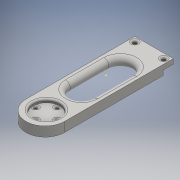
# Autodesk Inventor part: LowerArmPartAv2
Saved by Autodesk Inventor 2016 (Build 200138000, 138)
## iProperties
Created: 2015-10-06
Part Number: LowerArmPartAv2
Material: Generic
Document SubType Name: Modeling
Designer: alex
Density: 1 g/cm^3
Appearance: Default
Mass: 56.6565 g
Surface Area: 198.211 cm^2
Volume: 56.6565 cm^3
Author: alex
Autodesk Inventor part; units mm, degrees
ref_plane "YZ Plane" through (0, 0, 0) normal (1, 0, 0) x (0, 1, 0)
ref_plane "XZ Plane" through (0, 0, 0) normal (0, 1, 0) x (-1, 0, 0)
ref_plane "XY Plane" through (0, 0, 0) normal (0, 0, 1) x (1, 0, 0)
sketch "Sketch1" plane through (0, 0, 0) normal (0, 0, 1) x (1, 0, 0)
  line L0 (-20, 50) -> (20, 50)
  line L1 (20, 50) -> (20, -83)
  line L2 (20, -83) -> (-20, -83)
  line L3 (-20, -83) -> (-20, 50)
  point P0 (0, 0)
  dimension "d0" = 50
  dimension "d1" = 83
  dimension "d2" = 20
  dimension "d3" = 20
  constraints: 8 end point, 2 parallel, 1 horizontal, 1 perpendicular
  measures "d0" distance from line of point (0, 0) L0
  measures "d1" distance from line of point (0, 0) L2
  measures "d2" distance from line of point (0, 0) L3
  measures "d3" distance from line of point (0, 0) L1
extrude "Extrusion1" add sketch "Sketch1" along normal blind 10
sketch "Sketch6" plane through (0, 0, 10) normal (0, 0, 1) x (1, 0, 0)
  circle A0 centre (0, -61.75) radius 13.75
  arc A1 (-18, -63) -> (18, -63) centre (0, -63) ccw projected
  line L0 (18, 20) -> (18, -83) projected
  circle A2 centre (0, -50.5) radius 1.5
  circle A3 centre (-11.25, -61.75) radius 1.5
  circle A4 centre (0, -73) radius 1.5
  circle A5 centre (11.25, -61.75) radius 1.5
  line L1 (0, 0) -> (-53.5469, 0)
  dimension "d41" = 27.5
  dimension "d42" = 5.5
  dimension "d43" = 18
  dimension "d44" = 3
  dimension "d45" = 11.25
  dimension "d46" = 18
  dimension "d49" = 360
  constraints: 5 centre point, 2 end point, 1 horizontal, 9 other
  measures "d41" diameter of A0
  measures "d43" distance from line of L0 A0.centre
  measures "d44" diameter of A2
  measures "d45" distance of A0.centre A2.centre
  measures "d46" distance from line of L0 A2.centre
sketch "Sketch8" plane through (0, 0, 10) normal (0, 0, 1) x (1, 0, 0)
  circle A0 centre (0, -61.75) radius 13.75
  line L0 (-18, -83) -> (-18, 20) projected
  arc A1 (-18, -63) -> (18, -63) centre (0, -63) ccw projected
  line L1 (0, 0) -> (-37.1861, 0)
  dimension "d62" = 27.5
  dimension "d63" = 18
  dimension "d64" = 1.25
  constraints: 2 end point, 1 centre point, 1 horizontal
  measures "d62" diameter of A0
  measures "d63" distance from line of L0 A0.centre
  measures "d64" distance of A1.centre A0.centre
extrude "Extrusion8" cut sketch "Sketch8" against normal blind 3.5
fillet "Fillet12" radius 20 2 edges at (-20, -83, 5) (20, -83, 5)
sketch "Sketch10" plane through (0, 0, 10) normal (0, 0, 1) x (1, 0, 0)
  line L0 (0, 27) -> (0, -37) construction
  line L1 (-12, 15) -> (-12, -25)
  line L2 (12, -25) -> (12, 15)
  arc A0 (12, 15) -> (-12, 15) centre (0, 15) ccw
  arc A1 (-12, -25) -> (12, -25) centre (0, -25) ccw
  line L3 (20, 50) -> (-20, 50) projected
  line L4 (20, -63) -> (20, 50) projected
  line L5 (-20, 50) -> (-20, -63) projected
  point P0 (0, 0)
  point P1 (0, -5)
  dimension "d80" = 40
  dimension "d81" = 35
  dimension "d82" = 8
  dimension "d83" = 8
  constraints: 8 end point, 6 point on circle, 4 tangent, 2 centre point, 2 point on line, 1 midpoint, 1 parallel, 1 vertical
  measures "d80" distance of A1.centre A0.centre
  measures "d81" distance from line of L3 A0.centre
  measures "d82" distance between parallel lines of L4 L2
  measures "d83" distance between parallel lines of L5 L1
extrude "Extrusion10" cut sketch "Sketch10" against normal through all
sketch "Sketch11" plane through (0, 0, 10) normal (0, 0, 1) x (1, 0, 0)
  point P0 (0, 0)
extrude "Extrusion11" cut sketch "Sketch6" against normal through all contours A2 | A3 | A4 | A5
sketch "Sketch13" plane through (0, 0, 0) normal (0, 0, -1) x (-1, 0, 0)
  line L0 (20, -63) -> (20, 50) projected
  line L1 (-20, 50) -> (20, 50)
  line L2 (20, 50) -> (20, 39.5)
  line L3 (20, 39.5) -> (-20, 39.5)
  line L4 (-20, 39.5) -> (-20, 50)
  line L5 (20, 50) -> (-20, 50) projected
  point P0 (0, 0)
  dimension "d91" = 10.5
  dimension "d92" = 0
  dimension "d93" = 40
  constraints: 8 end point, 2 parallel, 1 horizontal, 1 perpendicular, 1 point on line
  measures "d91" distance between parallel lines of L3 L1
  measures "d92" distance between parallel lines of L5 L1
  measures "d93" distance between parallel lines of L0 L4
extrude "Extrusion13" cut sketch "Sketch13" against normal blind 5
sketch "Sketch14" plane through (0, 0, 5) normal (0, 0, -1) x (-1, 0, 0)
  circle A0 centre (-15, 45) radius 2
  line L0 (20, 39.5) -> (-20, 39.5) projected
  line L1 (-20, -63) -> (-20, 50) projected
  line L2 (0, 0) -> (0, 62.9691)
  circle A1 centre (15, 45) radius 2
  line L3 (-20, 50) -> (20, 50) projected
  dimension "d96" = 4
  dimension "d98" = 5
  dimension "d105" = 5
  constraints: 2 centre point, 2 end point, 1 symmetric about line, 1 vertical, 1 other
  measures "d96" diameter of A0
  measures "d98" distance from line of L1 A0.centre
  measures "d105" distance from line of L3 A0.centre
extrude "Extrusion14" cut sketch "Sketch14" against normal blind 10 contours A0 | A1
fillet "Fillet13" radius 5 8 edges at (0, -37, 10) (-12, -5, 10) (0, 27, 10) (12, -5, 10) (0, 27, 0) (-12, -5, 0) (0, -37, 0) (12, -5, 0)
fillet "Fillet14" radius 2 2 edges at (-13, 45, 10) (17, 45, 10)
fillet "Fillet15" radius 2 2 edges at (-13, 45, 5) (17, 45, 5)
fillet "Fillet16" radius 2 9 edges at (-13.75, -61.75, 10) (-1.5, -50.5, 6.5) (9.75, -61.75, 6.5) (-12.75, -61.75, 6.5) (-1.5, -73, 6.5) (9.75, -61.75, 0) (-1.5, -50.5, 0) (-12.75, -61.75, 0) (-1.5, -73, 0)
body "Solid1"
